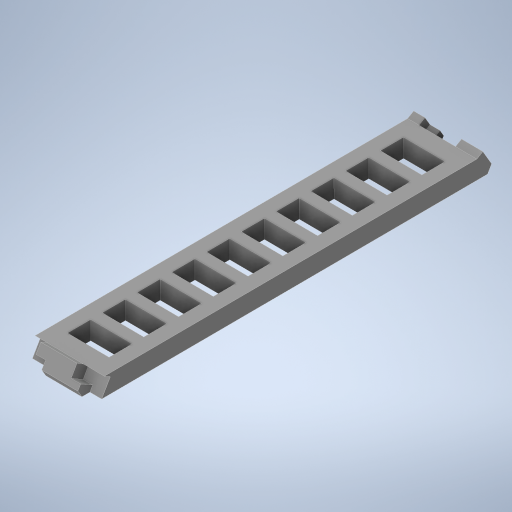
# Autodesk Inventor part: base
Saved by Autodesk Inventor 2024.3 (Build 283343000, 343)
## iProperties
Created: 2024-10-09
Part Number: base
Material: Generic
Document SubType Name: Modeling
Designer: pjcaa
Density: 1 g/cm^3
Appearance: Default(2)
Author: pjcaa
Autodesk Inventor part; units mm, degrees
ref_plane "YZ Plane" through (0, 0, 0) normal (1, 0, 0) x (0, 1, 0)
ref_plane "XZ Plane" through (0, 0, 0) normal (0, 1, 0) x (-1, 0, 0)
ref_plane "XY Plane" through (0, 0, 0) normal (0, 0, 1) x (1, 0, 0)
sketch "Sketch1" plane through (0, 0, 0) normal (0, 0, 1) x (1, 0, 0)
  line L0 (-85, -15) -> (85, -15)
  line L1 (85, -15) -> (85, 15)
  line L2 (85, 15) -> (-85, 15)
  line L3 (-85, 15) -> (-85, -15)
  line L4 (-85, -15) -> (85, 15) construction
  line L5 (85, -15) -> (-85, 15) construction
  point P0 (0, 0)
  dimension "d0" = 170
  dimension "d1" = 30
  constraints: 12 end point, 2 midpoint, 2 parallel, 1 horizontal, 1 perpendicular
  measures "d0" distance of L2.end L1.end
  measures "d1" distance of L1.end L0.end
extrude "Extrusion1" add sketch "Sketch1" along normal blind 8
sketch "Sketch2" plane through (-85, 15, 0) normal (0, 1, 0) x (1, 0, 0)
  line L0 (170, 0) -> (0, 0) construction
  line L1 (0, 0) -> (0, -8) construction
  line L2 (170, -8) -> (0, -8) construction
  line L3 (170, 0) -> (170, -8) construction
  line L4 (0, -8) -> (0, 0)
  line L5 (85, 0) -> (85, -8) construction
  line L6 (0, 0) -> (4.6188, -8)
  line L7 (0, -8) -> (4.6188, -8)
  line L8 (170, -8) -> (170, 0)
  line L9 (170, 0) -> (165.3812, -8)
  line L10 (170, -8) -> (165.3812, -8)
  point P0 (1.7321, 0)
  dimension "d7" = 30
  constraints: 14 end point, 2 collinear, 2 point on line, 1 midpoint, 1 symmetric about line
  measures "d7" angle of L1 L6
extrude "Extrusion3" cut sketch "Sketch2" against normal through all
sketch "Sketch3" plane through (-85, -15, 0) normal (-0.8660254, 0, 0.5) x (0.5, 0, 0.8660254)
  line L0 (9.2376, 0) -> (0, 0) construction
  line L1 (9.2376, 30) -> (9.2376, 0) construction
  line L2 (0, 30) -> (9.2376, 30) construction
  line L3 (0, 30) -> (0, 0) construction
  line L4 (85, 30) -> (0, 30) projected
  line L5 (9.2376, 30) -> (0, 30)
  line L6 (0, 30) -> (0, 20.7624)
  line L7 (9.2376, 30) -> (9.2376, 24.9)
  line L8 (9.2376, 24.9) -> (5.1, 24.9)
  line L9 (5.1, 24.9) -> (5.1, 20.7624)
  line L10 (5.1, 20.7624) -> (0, 20.7624)
  line L11 (9.2376, 0) -> (0, 0)
  line L12 (0, 0) -> (0, 5.1)
  line L13 (0, 5.1) -> (4.1376, 5.1)
  line L14 (4.1376, 5.1) -> (4.1376, 9.2376)
  line L15 (4.1376, 9.2376) -> (9.2376, 9.2376)
  line L16 (9.2376, 9.2376) -> (9.2376, 0)
  line L17 (9.2376, 24.9) -> (9.2376, 9.2376)
  line L18 (0, 5.1) -> (0, 20.7624)
  point P0 (42.5, 15)
  dimension "d17" = 5.1
  dimension "d18" = 5.1
  dimension "d19" = 5.1
  dimension "d20" = 5.1
  constraints: 28 end point, 5 horizontal, 5 perpendicular, 4 point on line, 3 collinear
  measures "d17" distance between parallel lines of L8 L2
  measures "d18" distance of L9.end L6.end
  measures "d19" distance between parallel lines of L0 L13
  measures "d20" distance of L14.end L15.end
extrude "Extrusion4" add sketch "Sketch3" along normal blind 3 contours L17 L15 L14 L13 L18 L10 L9 L8
sketch "Sketch5" plane through (-85, 5.7624, 0) normal (-0.8660254, 0, 0.5) x (0.5, 0, 0.8660254)
  line L0 (0, 0) -> (5.1, 0) projected
  line L1 (5.1, 0) -> (5.1, 4.1376) projected
  line L2 (5.1, 4.1376) -> (9.2376, 4.1376) projected
  line L3 (9.2376, 9.2376) -> (9.2376, 4.1376) projected
  line L4 (0, 9.2376) -> (9.2376, 9.2376) projected
  line L5 (0, 9.2376) -> (0, 0) projected
  line L6 (4.1376, -15.6624) -> (0, -15.6624) projected
  line L7 (0, -15.6624) -> (0, -20.7624) projected
  line L8 (9.2376, -20.7624) -> (0, -20.7624) projected
  line L9 (9.2376, -11.5248) -> (9.2376, -20.7624) projected
  line L10 (9.2376, -11.5248) -> (4.1376, -11.5248) projected
  line L11 (4.1376, -11.5248) -> (4.1376, -15.6624) projected
  point P0 (42.5, -5.7624)
extrude "Extrusion6" cut sketch "Sketch5" against normal blind 3
sketch "Sketch7" plane through (85, -15, 0) normal (0.8660254, 0, 0.5) x (0.5, 0, -0.8660254)
  line L0 (0, 0) -> (-9.2376, 0) construction
  line L1 (0, 0) -> (0, 30) construction
  line L2 (-9.2376, 30) -> (0, 30) construction
  line L3 (-9.2376, 0) -> (-9.2376, 30) construction
  line L4 (0, 0) -> (-9.2376, 0)
  line L5 (-9.2376, 9.2376) -> (-9.2376, 0)
  line L6 (-9.2376, 9.2376) -> (-4.3376, 9.2376)
  line L7 (-4.3376, 9.2376) -> (-4.3376, 4.9)
  line L8 (-4.3376, 4.9) -> (0, 4.9)
  line L9 (0, 0) -> (0, 4.9)
  line L10 (0, 30) -> (-9.2376, 30)
  line L11 (-9.2376, 30) -> (-9.2376, 25.1)
  line L12 (-9.2376, 25.1) -> (-4.9, 25.1)
  line L13 (-4.9, 25.1) -> (-4.9, 20.7624)
  line L14 (-4.9, 20.7624) -> (0, 20.7624)
  line L15 (0, 20.7624) -> (0, 30)
  point P0 (-42.5, 15)
  dimension "d34" = 4.9
  dimension "d35" = 4.9
  dimension "d36" = 4.9
  dimension "d37" = 4.9
  constraints: 24 end point, 7 perpendicular, 4 point on line, 3 collinear, 2 horizontal, 1 vertical
  measures "d34" distance between parallel lines of L0 L8
  measures "d35" distance of L5.start L6.end
  measures "d36" distance of L13.end L14.end
  measures "d37" distance between parallel lines of L2 L12
extrude "Extrusion8" add sketch "Sketch7" along normal blind 3
sketch "Sketch9" plane through (85, -10.1, 0) normal (0.8660254, 0, 0.5) x (0.5, 0, -0.8660254)
  line L0 (0, 15.8624) -> (-4.9, 15.8624) projected
  line L1 (-4.9, 15.8624) -> (-4.9, 20.2) projected
  line L2 (-4.9, 20.2) -> (-9.2376, 20.2) projected
  line L3 (-9.2376, 4.3376) -> (-9.2376, 20.2) projected
  line L4 (-9.2376, 4.3376) -> (-4.3376, 4.3376) projected
  line L5 (-4.3376, 4.3376) -> (-4.3376, 0) projected
  line L6 (-4.3376, 0) -> (0, 0) projected
  line L7 (0, 0) -> (0, 15.8624) projected
  point P0 (-42.5, 10.1)
extrude "Extrusion10" cut sketch "Sketch9" against normal blind 3
sketch "Sketch6" plane through (-81.5359, -15, 0) normal (0, -1, 0) x (1, 0, 0)
  line L0 (-3.9934, 5.0833) -> (1.2028, 2.0833) construction
  line L1 (-6.0622, 1.5) -> (-3.9934, 5.0833) construction
  line L2 (-3.4641, 0) -> (-6.0622, 1.5) construction
  line L3 (0, 0) -> (-3.4641, 0) construction
  line L4 (0, 0) -> (1.2028, 2.0833) construction
  line L5 (1.1547, 8) -> (-1.4434, 9.5) construction
  line L6 (-3.9934, 5.0833) -> (-1.4434, 9.5) construction
  line L7 (-3.9934, 5.0833) -> (1.2028, 2.0833) construction
  line L8 (1.2028, 2.0833) -> (3.7528, 6.5) construction
  line L9 (1.1547, 8) -> (3.7528, 6.5) construction
  line L10 (-3.4641, 0) -> (-6.0622, 1.5)
  line L11 (-5.1962, 3) -> (-6.0622, 1.5)
  line L12 (-3.4641, 0) -> (-5.1962, 3)
  line L13 (166.9652, 5.2565) -> (161.769, 2.2565) construction
  line L14 (3.7528, 6.5) -> (0, 0) construction
  line L15 (0, 0) -> (166.5359, 0) construction
  line L16 (166.5359, 0) -> (169.134, 1.5) construction
  line L17 (164.5152, 9.5) -> (169.134, 1.5) construction
  line L18 (161.9171, 8) -> (164.5152, 9.5) construction
  line L19 (1.1547, 8) -> (161.9171, 8) construction
  line L20 (1.1547, 8) -> (3.7528, 6.5) construction
  line L21 (166.5359, 0) -> (169.134, 1.5)
  line L22 (169.134, 1.5) -> (168.2679, 3)
  line L23 (168.2679, 3) -> (166.5359, 0)
  point P0 (81.5359, 0)
  dimension "d23" = 30
  dimension "d40" = 30
  constraints: 13 end point, 2 point on line, 1 perpendicular
  measures "d23" angle of L12 L2
  measures "d40" angle of L23 L16
extrude "Extrusion7" cut sketch "Sketch6" against normal through all
sketch "Sketch11" plane through (0, 0, 8) normal (0, 0, 1) x (1, 0, 0)
  line L0 (80.3812, -15) -> (80.3812, -5.7624) construction
  line L1 (80.3812, -5.7624) -> (80.3812, 10.1) construction
  line L2 (80.3812, 10.1) -> (80.3812, 15) construction
  line L3 (80.3812, 15) -> (-80.3812, 15) construction
  line L4 (-80.3812, 15) -> (-80.3812, 9.9) construction
  line L5 (-80.3812, 9.9) -> (-80.3812, -5.7624) construction
  line L6 (-80.3812, -5.7624) -> (-80.3812, -15) construction
  line L7 (-80.3812, -15) -> (80.3812, -15) construction
  line L8 (-62.3812, -9) -> (-72.3812, -9)
  line L9 (-72.3812, -9) -> (-72.3812, 9)
  line L10 (-72.3812, 9) -> (-62.3812, 9)
  line L11 (-62.3812, 9) -> (-62.3812, -9)
  line L12 (-47.3812, -9) -> (-57.3812, -9)
  line L13 (-57.3812, -9) -> (-57.3812, 9)
  line L14 (-57.3812, 9) -> (-47.3812, 9)
  line L15 (-47.3812, 9) -> (-47.3812, -9)
  line L16 (-32.3812, -9) -> (-42.3812, -9)
  line L17 (-42.3812, -9) -> (-42.3812, 9)
  line L18 (-42.3812, 9) -> (-32.3812, 9)
  line L19 (-32.3812, 9) -> (-32.3812, -9)
  line L20 (-17.3812, -9) -> (-27.3812, -9)
  line L21 (-27.3812, -9) -> (-27.3812, 9)
  line L22 (-27.3812, 9) -> (-17.3812, 9)
  line L23 (-17.3812, 9) -> (-17.3812, -9)
  line L24 (-2.3812, -9) -> (-12.3812, -9)
  line L25 (-12.3812, -9) -> (-12.3812, 9)
  line L26 (-12.3812, 9) -> (-2.3812, 9)
  line L27 (-2.3812, 9) -> (-2.3812, -9)
  line L28 (12.6188, -9) -> (2.6188, -9)
  line L29 (2.6188, -9) -> (2.6188, 9)
  line L30 (2.6188, 9) -> (12.6188, 9)
  line L31 (12.6188, 9) -> (12.6188, -9)
  line L32 (27.6188, -9) -> (17.6188, -9)
  line L33 (17.6188, -9) -> (17.6188, 9)
  line L34 (17.6188, 9) -> (27.6188, 9)
  line L35 (27.6188, 9) -> (27.6188, -9)
  line L36 (42.6188, -9) -> (32.6188, -9)
  line L37 (32.6188, -9) -> (32.6188, 9)
  line L38 (32.6188, 9) -> (42.6188, 9)
  line L39 (42.6188, 9) -> (42.6188, -9)
  line L40 (57.6188, -9) -> (47.6188, -9)
  line L41 (47.6188, -9) -> (47.6188, 9)
  line L42 (47.6188, 9) -> (57.6188, 9)
  line L43 (57.6188, 9) -> (57.6188, -9)
  line L44 (72.6188, -9) -> (62.6188, -9)
  line L45 (62.6188, -9) -> (62.6188, 9)
  line L46 (62.6188, 9) -> (72.6188, 9)
  line L47 (72.6188, 9) -> (72.6188, -9)
  point P0 (0, 0)
  point P1 (-72.3812, 0)
  point P2 (-80.3812, 12.45)
  point P3 (-57.3812, 0)
  point P4 (-42.3812, 0)
  point P5 (-27.3812, 0)
  point P6 (-12.3812, 0)
  point P7 (2.6188, 0)
  point P8 (17.6188, 0)
  point P9 (32.6188, 0)
  point P10 (47.6188, 0)
  point P11 (62.6188, 0)
  dimension "d53" = 10
  dimension "d54" = 18
  dimension "d55" = 8
  dimension "d58" = 15
  constraints: 80 end point, 2 horizontal, 2 midpoint, 2 parallel, 1 horizontal alignment, 1 perpendicular, 81 other
  measures "d53" distance of L9.end L10.end
  measures "d54" distance of L8.end L9.end
  measures "d55" horizontal distance of point (-80.381, 12.45) L9.end
  measures "d58" distance of L8.start L12.start
extrude "Extrusion12" cut sketch "Sketch11" against normal through all
body "Solid1"
